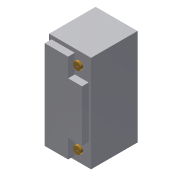
# Autodesk Inventor part: 17-0028-0034
Saved by Autodesk Inventor 2016 SP2 (Build 200236200, 236)
## iProperties
Category: IOP
Company: Universiteit van Amsterdam
Created: 2017-11-20
Part Number: 17-0028-0034
Material: ABS Plastic
Document SubType Name: Modeling
Designer: Daan Giesen
Density: 1.06 g/cm^3
Appearance: Smooth - White
Project: Digital PID Loop
Cost Center: 17-0028
User Status: Work in Progress
Authority: Reichsöllner, Lukas
Description: Battery
Author: Daan Giesen
Title: Digital PID Loop
Revision Number: A
Autodesk Inventor part; units mm, degrees
ref_plane "YZ Plane" through (0, 0, 0) normal (1, 0, 0) x (0, 1, 0)
ref_plane "XZ Plane" through (0, 0, 0) normal (0, 1, 0) x (-1, 0, 0)
ref_plane "XY Plane" through (0, 0, 0) normal (0, 0, 1) x (1, 0, 0)
sketch "Sketch1" plane through (0, 0, 0) normal (0, 0, 1) x (1, 0, 0)
  line L0 (0, 158.9) -> (0, -158.9) construction
  line L1 (-125.3, 0) -> (125.3, 0) construction
  line L2 (89.5, -113.5) -> (-89.5, -113.5)
  line L3 (-89.5, -113.5) -> (-89.5, 113.5)
  line L4 (-89.5, 113.5) -> (89.5, 113.5)
  line L5 (89.5, 113.5) -> (89.5, -113.5)
  line L6 (89.5, -113.5) -> (-89.5, 113.5) construction
  line L7 (-89.5, -113.5) -> (89.5, 113.5) construction
  point P0 (0, 0)
  dimension "d4" = 227
  dimension "d5" = 179
  constraints: 12 end point, 2 midpoint, 2 parallel, 1 horizontal, 1 perpendicular
  measures "d4" distance of L2.end L3.end
  measures "d5" distance of L3.end L4.end
extrude "Extrusion3" add sketch "Sketch1" along normal mid plane 412
sketch "Sketch2" plane through (-89.5, -113.5, 206) normal (0, -1, 0) x (1, 0, 0)
  line L0 (179, -412) -> (179, 0) projected
  line L1 (0, 0) -> (179, 0) projected
  line L2 (0, 0) -> (0, -412) projected
  line L3 (179, -412) -> (0, -412) projected
  line L4 (109.5, -16) -> (10, -16)
  line L5 (10, -16) -> (10, -396)
  line L6 (10, -396) -> (109.5, -396)
  line L7 (109.5, -396) -> (109.5, -16)
  line L8 (109.5, -16) -> (10, -396) construction
  line L9 (10, -16) -> (109.5, -396) construction
  line L10 (169, -96) -> (109.5, -96)
  line L11 (109.5, -96) -> (109.5, -316)
  line L12 (109.5, -316) -> (169, -316)
  line L13 (169, -316) -> (169, -96)
  line L14 (169, -96) -> (109.5, -316) construction
  line L15 (109.5, -96) -> (169, -316) construction
  point P0 (89.5, -206)
  point P1 (59.75, -206)
  point P2 (139.25, -206)
  point P3 (59.75, -206)
  point P4 (139.25, -206)
  dimension "d8" = 220
  dimension "d9" = 380
  dimension "d10" = 10
  dimension "d11" = 10
  dimension "d12" = 20
  constraints: 24 end point, 6 midpoint, 4 parallel, 2 horizontal, 2 horizontal alignment, 2 perpendicular, 1 point on line
  measures "d8" distance of L12.end L10.start
  measures "d9" distance of L4.end L5.end
  measures "d10" distance between parallel lines of L2 L5
  measures "d11" distance between parallel lines of L0 L13
  measures "d12" distance from line of L11 point (89.5, -206)
extrude "Extrusion4" cut sketch "Sketch2" against normal blind 28.5
sketch "Sketch3" plane through (-89.5, -85, 206) normal (0, -1, 0) x (1, 0, 0)
  circle A0 centre (129.1, -361.5) radius 16.2143
  circle A1 centre (129.1, -50.5) radius 16.2143
  line L0 (179, -412) -> (0, -412) projected
  line L1 (0, 0) -> (179, 0) projected
  line L2 (89.5, 82.4) -> (89.5, -494.4) projected
  point P0 (89.5, -206)
  dimension "d17" = 311
  dimension "d18" = 50.5
  dimension "d20" = 50.5
  dimension "d21" = 39.6
  constraints: 2 centre point, 1 equal radius, 1 vertical alignment
  measures "d17" distance of A1.centre A0.centre
  measures "d18" distance from line of A0.centre L0
  measures "d20" distance from line of L1 A1.centre
  measures "d21" distance from line of A0.centre L2
extrude "Extrusion5" add sketch "Sketch3" along normal blind 10.5
sketch "Sketch4" plane through (39.6, -95.5, -155.5) normal (0, -1, 0) x (1, 0, 0)
  circle A0 centre (0, 0) radius 16.2143 projected
  circle A1 centre (0, 311) radius 16.2143 projected
  line L0 (49.9, 361.5) -> (49.9, -50.5) projected
  line L1 (-129.1, 361.5) -> (49.9, 361.5) projected
  line L2 (-129.1, -50.5) -> (-129.1, 361.5) projected
  line L3 (49.9, -50.5) -> (-129.1, -50.5) projected
  line L4 (-19.6, 265.5) -> (-19.6, 345.5) projected
  line L5 (39.9, 265.5) -> (-19.6, 265.5) projected
  line L6 (39.9, 45.5) -> (39.9, 265.5) projected
  line L7 (-19.6, 45.5) -> (39.9, 45.5) projected
  line L8 (-19.6, -34.5) -> (-19.6, 45.5) projected
  line L9 (-119.1, -34.5) -> (-19.6, -34.5) projected
  line L10 (-119.1, 345.5) -> (-119.1, -34.5) projected
  line L11 (-19.6, 345.5) -> (-119.1, 345.5) projected
  point P0 (-39.6, 155.5)
  constraints: 2 coincident
hole "Hole1" at (39.6, -95.5, -155.5) at (39.6, -95.5, 155.5) direction (0, 1, 0) diameter 6.647 depth 10 tip angle 118 thread size "M8x1.25" class "6H" standard "ISO Metric profile"
equation "\"d18\" = d20"
body "Solid3"
